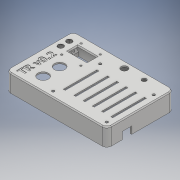
# Autodesk Inventor part: TestingRemoteHousing
Saved by Autodesk Inventor 2018.3 (Build 223284000, 284)
## iProperties
Created: 2019-03-25
Part Number: TestingRemoteHousing
Material: Generic
Document SubType Name: Modeling
Designer: matth
Density: 1 g/cm^3
Appearance: Default
Author: matth
Autodesk Inventor part; units mm, degrees
ref_plane "YZ Plane" through (0, 0, 0) normal (1, 0, 0) x (0, 1, 0)
ref_plane "XZ Plane" through (0, 0, 0) normal (0, 1, 0) x (-1, 0, 0)
ref_plane "XY Plane" through (0, 0, 0) normal (0, 0, 1) x (1, 0, 0)
sketch "Sketch1" plane through (0, 0, 0) normal (0, 0, 1) x (1, 0, 0)
  line L0 (-6.9712, 4.0639) -> (131.4288, 4.0639)
  line L1 (138.4288, -2.9361) -> (138.4288, -90.5361)
  line L2 (131.4288, -97.5361) -> (-6.9712, -97.5361)
  line L3 (-13.9712, -90.5361) -> (-13.9712, -2.9361)
  arc A0 (-6.9712, 4.0639) -> (-13.9712, -2.9361) centre (-6.9712, -2.9361) ccw
  arc A1 (-13.9712, -90.5361) -> (-6.9712, -97.5361) centre (-6.9712, -90.5361) ccw
  arc A2 (131.4288, -97.5361) -> (138.4288, -90.5361) centre (131.4288, -90.5361) ccw
  arc A3 (138.4288, -2.9361) -> (131.4288, 4.0639) centre (131.4288, -2.9361) ccw
  circle A4 centre (103.4288, -5.9361) radius 3.43
  circle A5 centre (130.4288, -89.5361) radius 2
  circle A6 centre (49.2288, -89.5361) radius 2
  circle A7 centre (49.2288, -18.3361) radius 2
  circle A8 centre (130.4288, -18.3361) radius 2
  circle A9 centre (8.0288, -5.9361) radius 1.5
  circle A10 centre (36.9848, -5.9361) radius 1.5
  circle A11 centre (8.0288, -35.4001) radius 1.5
  circle A12 centre (36.9848, -35.4001) radius 1.5
  circle A13 centre (22.0288, -52.5361) radius 8
  circle A14 centre (22.0288, -77.5361) radius 8
  line L4 (-7.9712, -7.9361) -> (0.2288, -7.9361)
  line L5 (0.2288, -7.9361) -> (0.2288, -16.1361)
  line L6 (0.2288, -16.1361) -> (-7.9712, -16.1361)
  line L7 (-7.9712, -16.1361) -> (-7.9712, -7.9361)
  line L8 (-7.9712, -20.8361) -> (0.2288, -20.8361)
  line L9 (0.2288, -20.8361) -> (0.2288, -29.0361)
  line L10 (0.2288, -29.0361) -> (-7.9712, -29.0361)
  line L11 (-7.9712, -29.0361) -> (-7.9712, -20.8361)
  circle A15 centre (73.4288, -5.9361) radius 5
  line L12 (8.0288, -26.0021) -> (36.9848, -26.0021)
  line L13 (36.9848, -26.0021) -> (36.9848, -11.0021)
  line L14 (36.9848, -11.0021) -> (8.0288, -11.0021)
  line L15 (8.0288, -11.0021) -> (8.0288, -26.0021)
  line L16 (54.5635, -28.5361) -> (57.5635, -28.5361)
  line L17 (57.5635, -28.5361) -> (57.5635, -79.5361)
  line L18 (57.5635, -79.5361) -> (54.5635, -79.5361)
  line L19 (54.5635, -79.5361) -> (54.5635, -28.5361)
  line L20 (70.5888, -79.5361) -> (73.5888, -79.5361)
  line L21 (73.5888, -79.5361) -> (73.5888, -28.5361)
  line L22 (73.5888, -28.5361) -> (70.5888, -28.5361)
  line L23 (70.5888, -28.5361) -> (70.5888, -79.5361)
  line L24 (84.5588, -28.5361) -> (87.5588, -28.5361)
  line L25 (87.5588, -28.5361) -> (87.5588, -79.5361)
  line L26 (87.5588, -79.5361) -> (84.5588, -79.5361)
  line L27 (84.5588, -79.5361) -> (84.5588, -28.5361)
  line L28 (98.5288, -28.5361) -> (101.5288, -28.5361)
  line L29 (101.5288, -28.5361) -> (101.5288, -79.5361)
  line L30 (101.5288, -79.5361) -> (98.5288, -79.5361)
  line L31 (98.5288, -79.5361) -> (98.5288, -28.5361)
  line L32 (112.4288, -28.5361) -> (115.4288, -28.5361)
  line L33 (115.4288, -28.5361) -> (115.4288, -79.5361)
  line L34 (115.4288, -79.5361) -> (112.4288, -79.5361)
  line L35 (112.4288, -79.5361) -> (112.4288, -28.5361)
  line L36 (126.4688, -28.5361) -> (129.4688, -28.5361)
  line L37 (129.4688, -28.5361) -> (129.4688, -79.5361)
  line L38 (129.4688, -79.5361) -> (126.4688, -79.5361)
  line L39 (126.4688, -79.5361) -> (126.4688, -28.5361)
  point P0 (0, 0)
  point P1 (138.4288, -97.5361)
  point P2 (138.4288, 4.0639)
  point P3 (-13.9712, -97.5361)
  dimension "d0" = 152.4
  dimension "d1" = 101.6
  dimension "d2" = 7
  dimension "d3" = 6.86
  dimension "d4" = 10
  dimension "d5" = 35
  dimension "d6" = 4
  dimension "d7" = 4
  dimension "d8" = 4
  dimension "d9" = 81.2
  dimension "d10" = 8
  dimension "d11" = 0
  dimension "d12" = 71.2
  dimension "d13" = 4
  dimension "d14" = 8
  dimension "d15" = 3
  dimension "d16" = 3
  dimension "d17" = 28.956
  dimension "d18" = 22
  dimension "d19" = 3
  dimension "d20" = 29.464
  dimension "d21" = 3
  dimension "d22" = 16
  dimension "d23" = 16
  dimension "d24" = 20
  dimension "d25" = 63.2
  dimension "d26" = 36
  dimension "d27" = 36
  dimension "d28" = 25
  dimension "d29" = 10
  dimension "d30" = 0
  dimension "d31" = 8.2
  dimension "d32" = 8.2
  dimension "d33" = 6
  dimension "d34" = 12
  dimension "d35" = 8.2
  dimension "d36" = 10
  dimension "d37" = 10
  dimension "d38" = 65
  dimension "d39" = 0
  dimension "d40" = 28.956
  dimension "d41" = 15
  dimension "d42" = 9.398
  dimension "d43" = 0
  dimension "d44" = 3
  dimension "d45" = 51
  dimension "d46" = 10.2
  dimension "d47" = 3
  dimension "d48" = 51
  dimension "d49" = 3
  dimension "d50" = 51
  dimension "d51" = 3
  dimension "d52" = 51
  dimension "d53" = 3
  dimension "d54" = 51
  dimension "d55" = 3
  dimension "d56" = 51
  dimension "d57" = 21.36
  dimension "d58" = 35.33
  dimension "d59" = 49.3
  dimension "d60" = 63.2
  dimension "d61" = 80.24
  dimension "d112" = 8.2
  dimension "d113" = 0
  constraints: 80 end point, 20 parallel, 16 centre point, 10 horizontal, 10 perpendicular, 10 point on line, 8 point on circle, 8 tangent, 3 equal radius
  measures "d0" distance of point (138.429, -97.536) point (-13.971, -97.536)
  measures "d1" distance of point (138.429, 4.064) point (138.429, -97.536)
  measures "d2" radius of A0
  measures "d3" diameter of A4
  measures "d4" distance from line of L0 A4.centre
  measures "d5" distance from line of L1 A4.centre
  measures "d6" diameter of A5
  measures "d7" diameter of A6
  measures "d8" diameter of A7
  measures "d9" distance of A6.centre A5.centre
  measures "d10" distance from line of L1 A5.centre
  measures "d11" horizontal distance of A7.centre A6.centre
  measures "d12" distance of A6.centre A7.centre
  measures "d13" diameter of A8
  measures "d14" distance from line of L2 A5.centre
  measures "d15" diameter of A9
  measures "d16" diameter of A10
  measures "d17" distance of A10.centre A9.centre
  measures "d18" distance from line of L3 A9.centre
  measures "d19" diameter of A11
  measures "d20" distance of A9.centre A11.centre
  measures "d21" diameter of A12
  measures "d22" diameter of A13
  measures "d23" diameter of A14
  measures "d24" distance from line of L2 A14.centre
  measures "d25" distance from line of A6.centre L3
  measures "d26" distance from line of L3 A14.centre
  measures "d27" distance from line of A13.centre L3
  measures "d28" distance of A14.centre A13.centre
  measures "d29" distance from line of L0 A9.centre
  measures "d30" vertical distance of A11.centre A12.centre
  measures "d31" distance of L5.end L6.end
  measures "d32" distance of L4.end L5.end
  measures "d33" distance between parallel lines of L3 L7
  measures "d34" distance between parallel lines of L0 L4
  measures "d35" distance of L8.end L9.end
  measures "d36" diameter of A15
  measures "d37" distance from line of A15.centre L0
  measures "d38" distance from line of L1 A15.centre
  measures "d39" vertical distance of A8.centre A7.centre
  measures "d40" distance of L14.end L13.end
  measures "d41" distance of L12.end L13.end
  measures "d42" distance from line of L12 A11.centre
  measures "d43" distance from line of A10.centre L13
  measures "d44" distance of L17.end L18.end
  measures "d45" distance of L16.end L17.end
  measures "d46" distance from line of A7.centre L16
  measures "d47" distance of L22.end L21.end
  measures "d48" distance of L21.end L20.end
  measures "d49" distance of L25.end L26.end
  measures "d50" distance of L24.end L25.end
  measures "d51" distance of L29.end L30.end
  measures "d52" distance of L28.end L29.end
  measures "d53" distance of L33.end L34.end
  measures "d54" distance of L32.end L33.end
  measures "d55" distance of L37.end L38.end
  measures "d56" distance of L36.end L37.end
  measures "d57" distance from line of L23 A7.centre
  measures "d58" distance from line of A7.centre L27
  measures "d59" distance from line of L31 A7.centre
  measures "d60" distance from line of A7.centre L35
  measures "d61" distance from line of A7.centre L37
  measures "d112" distance of L9.end L10.end
  measures "d113" distance between parallel lines of L7 L11
extrude "Extrusion1" add sketch "Sketch1" along normal blind 2
chamfer "Chamfer1" distance 1 distance2 2 1 edges at (36.9848, -18.5021, 2) measured on face at (37.4848, -18.5021, 2)
chamfer "Chamfer2" distance 1 distance2 2 2 edges at (37.4848, -11.0021, 2) (22.5068, -11.0021, 2) measured on face at (37.4848, -10.5021, 2) measured on face at (22.5068, -10.5021, 2)
chamfer "Chamfer3" distance 1 distance2 2 2 edges at (8.0288, -10.5021, 2) (8.0288, -18.5021, 2) measured on face at (7.5288, -18.5021, 2) measured on face at (7.5288, -10.5021, 2)
chamfer "Chamfer4" distance 1 distance2 2 3 edges at (7.5289, -26.0021, 2) (22.5068, -26.0021, 2) (37.4848, -26.0021, 2) measured on face at (37.4848, -26.5021, 2) measured on face at (22.5068, -26.5021, 2) measured on face at (7.5289, -26.5021, 2)
chamfer "Chamfer5" distance 1 distance2 2 8 edges at (-13.9712, -46.7361, 2) (-11.9209, -95.4858, 2) (62.2288, -97.5361, 2) (136.3786, -95.4858, 2) (138.4288, -46.7361, 2) (136.3786, 2.0136, 2) (62.2288, 4.0639, 2) (-11.9209, 2.0136, 2) measured on face at (136.025, 1.6601, 2) measured on face at (62.2288, -97.0361, 2) measured on face at (62.2288, 3.5639, 2) measured on face at (-11.5674, -95.1323, 2) measured on face at (-11.5674, 1.6601, 2) measured on face at (137.9288, -46.7361, 2) measured on face at (136.025, -95.1323, 2) measured on face at (-13.4712, -46.7361, 2)
sketch "Sketch2" plane through (0, 0, 0) normal (0, 0, -1) x (-1, 0, 0)
  line L0 (6.9712, -97.5361) -> (-131.4288, -97.5361) projected
  arc A0 (6.9712, -97.5361) -> (13.9712, -90.5361) centre (6.9712, -90.5361) ccw projected
  line L1 (13.9712, -2.9361) -> (13.9712, -90.5361) projected
  arc A1 (13.9712, -2.9361) -> (6.9712, 4.0639) centre (6.9712, -2.9361) ccw projected
  line L2 (-131.4288, 4.0639) -> (6.9712, 4.0639) projected
  arc A2 (-131.4288, 4.0639) -> (-138.4288, -2.9361) centre (-131.4288, -2.9361) ccw projected
  line L3 (-138.4288, -90.5361) -> (-138.4288, -2.9361) projected
  arc A3 (-138.4288, -90.5361) -> (-131.4288, -97.5361) centre (-131.4288, -90.5361) ccw projected
  line L4 (-131.4288, -95.5361) -> (6.9712, -95.5361)
  arc A4 (6.9712, -95.5361) -> (11.9712, -90.5361) centre (6.9712, -90.5361) ccw
  line L5 (11.9712, -90.5361) -> (11.9712, -2.9361)
  arc A5 (11.9712, -2.9361) -> (6.9712, 2.0639) centre (6.9712, -2.9361) ccw
  line L6 (6.9712, 2.0639) -> (-131.4288, 2.0639)
  arc A6 (-131.4288, 2.0639) -> (-136.4288, -2.9361) centre (-131.4288, -2.9361) ccw
  line L7 (-136.4288, -2.9361) -> (-136.4288, -90.5361)
  arc A7 (-136.4288, -90.5361) -> (-131.4288, -95.5361) centre (-131.4288, -90.5361) ccw
  point P0 (0, 0)
  dimension "d79" = 2
  constraints: 8 end point, 8 point on circle, 4 centre point, 7 other
  measures "d79" distance between parallel lines of L0 L4
extrude "Extrusion2" add sketch "Sketch2" along normal blind 25
sketch "Sketch3" plane through (0, 0, -25) normal (0, 0, -1) x (-1, 0, 0)
  line L0 (-131.4288, 2.0639) -> (6.9712, 2.0639) projected
  arc A0 (-131.4288, 2.0639) -> (-136.4288, -2.9361) centre (-131.4288, -2.9361) ccw projected
  line L1 (-136.4288, -90.5361) -> (-136.4288, -2.9361) projected
  arc A1 (-136.4288, -90.5361) -> (-131.4288, -95.5361) centre (-131.4288, -90.5361) ccw projected
  line L2 (6.9712, -95.5361) -> (-131.4288, -95.5361) projected
  arc A2 (6.9712, -95.5361) -> (11.9712, -90.5361) centre (6.9712, -90.5361) ccw projected
  line L3 (11.9712, -2.9361) -> (11.9712, -90.5361) projected
  arc A3 (11.9712, -2.9361) -> (6.9712, 2.0639) centre (6.9712, -2.9361) ccw projected
  line L4 (3.9712, -5.9361) -> (-128.4288, -5.9361)
  line L5 (-128.4288, -5.9361) -> (-128.4288, -87.5361)
  line L6 (-128.4288, -87.5361) -> (3.9712, -87.5361)
  line L7 (3.9712, -87.5361) -> (3.9712, -5.9361)
  line L8 (-128.4288, -5.9361) -> (-128.4288, 2.0639)
  line L9 (-128.4288, -5.9361) -> (-136.4288, -5.9361)
  line L10 (3.9712, -5.9361) -> (3.9712, 2.0639)
  line L11 (3.9712, -5.9361) -> (11.9712, -5.9361)
  line L12 (-128.4288, -87.5361) -> (11.9712, -87.5361)
  line L13 (11.9712, -90.5361) -> (11.9712, -2.9361) projected
  line L14 (3.9712, -5.9361) -> (3.9712, -95.5361)
  line L15 (-131.4288, -95.5361) -> (6.9712, -95.5361) projected
  line L16 (-128.4288, -87.5361) -> (-136.4288, -87.5361)
  line L17 (-136.4288, -2.9361) -> (-136.4288, -90.5361) projected
  line L18 (-128.4288, -87.5361) -> (-128.4288, -95.5361)
  point P0 (0, 0)
  dimension "d82" = 8
  constraints: 24 end point, 12 point on line, 4 perpendicular, 2 vertical, 3 other
  measures "d82" distance between parallel lines of L0 L4
extrude "Extrusion3" add sketch "Sketch3" against normal blind 14 contours L0 L8 L9 L1 A0 | L0 A3 L3 L11 L10 | L11 L3 L12 L7 | L18 L2 A1 L1 L16 | L12 L3 A2 L2 L14
chamfer "Chamfer6" distance 8 angle 45 3 edges at (128.4288, -91.5361, -11) (128.4288, -1.9361, -11) (-3.9712, -46.7361, -11)
sketch "Sketch4" plane through (0, 0, -25) normal (0, 0, -1) x (-1, 0, 0)
  circle A0 centre (-131.4288, -90.5361) radius 1.75
  line L0 (-138.4288, -2.9361) -> (-138.4288, -90.5361) projected
  line L1 (-131.4288, -97.5361) -> (6.9712, -97.5361) projected
  circle A1 centre (-131.4288, -2.9361) radius 1.75
  line L2 (6.9712, 4.0639) -> (-131.4288, 4.0639) projected
  circle A2 centre (6.9712, -2.9361) radius 1.75
  line L3 (13.9712, -90.5361) -> (13.9712, -2.9361) projected
  circle A3 centre (6.9712, -90.5361) radius 1.75
  point P0 (0, 0)
  dimension "d88" = 3.5
  dimension "d89" = 7
  dimension "d90" = 7
  dimension "d91" = 3.5
  dimension "d92" = 7
  dimension "d93" = 7
  dimension "d94" = 3.5
  dimension "d95" = 7
  dimension "d96" = 7
  dimension "d97" = 3.5
  dimension "d98" = 7
  dimension "d99" = 7
  constraints: 4 centre point
  measures "d88" diameter of A0
  measures "d89" distance from line of L0 A0.centre
  measures "d90" distance from line of L1 A0.centre
  measures "d91" diameter of A1
  measures "d92" distance from line of L0 A1.centre
  measures "d93" distance from line of L2 A1.centre
  measures "d94" diameter of A2
  measures "d95" distance from line of L3 A2.centre
  measures "d96" distance from line of L2 A2.centre
  measures "d97" diameter of A3
  measures "d98" distance from line of L1 A3.centre
  measures "d99" distance from line of L3 A3.centre
extrude "Extrusion4" cut sketch "Sketch4" against normal blind 12
sketch "Sketch5" plane through (138.4288, -90.5361, 0) normal (1, 0, 0) x (0, 0, -1)
  line L0 (-2, -1) -> (-2, 3) projected
  line L1 (-2, 70.2) -> (-2, 74.2) projected
  line L2 (14, 16.5909) -> (25, 16.5909)
  line L3 (25, 16.5909) -> (25, 30.5909)
  line L4 (25, 30.5909) -> (14, 30.5909)
  line L5 (14, 30.5909) -> (14, 16.5909)
  line L6 (-2, 87.6) -> (-2, 0) projected
  line L7 (25, 87.6) -> (25, 0) projected
  point P0 (0, 90.5361)
  point P1 (-2, 1)
  point P2 (-2, 72.2)
  dimension "d102" = 11
  dimension "d103" = 14
  dimension "d105" = 0
  constraints: 8 end point, 2 midpoint, 2 parallel, 1 horizontal, 1 perpendicular
  measures "d102" distance of L4.end L3.end
  measures "d103" distance of L3.end L2.end
  measures "d105" distance between parallel lines of L7 L3
extrude "Extrusion5" cut sketch "Sketch5" against normal blind 10
sketch "Sketch6" plane through (0, 0, -25) normal (0, 0, -1) x (-1, 0, 0)
  line L0 (3.9712, 2.0639) -> (3.9712, -95.5361) projected
  line L1 (13.9712, -90.5361) -> (13.9712, -2.9361) projected
  line L2 (3.9712, -87.5361) -> (11.9712, -87.5361)
  line L3 (11.9712, -90.5361) -> (11.9712, -2.9361) projected
  line L4 (11.9712, -5.9361) -> (3.9712, -5.9361)
  line L5 (-128.4288, -87.5361) -> (-136.4288, -87.5361) projected
  line L6 (-136.4288, -5.9361) -> (-128.4288, -5.9361) projected
  line L7 (3.9712, -87.5361) -> (3.9712, -5.9361)
  line L8 (11.9712, -5.9361) -> (11.9712, -87.5361)
  point P0 (0, 0)
  dimension "d108" = 0
  dimension "d109" = 0
  constraints: 8 end point, 3 point on line, 1 collinear, 1 horizontal, 1 perpendicular, 1 vertical
  measures "d108" distance between parallel lines of L5 L2
  measures "d109" distance between parallel lines of L6 L4
extrude "Extrusion6" cut sketch "Sketch6" against normal up to surface (25 mm away)
sketch "Sketch7" plane through (0, 0, 2) normal (0, 0, 1) x (1, 0, 0)
  line L0 (-7.9712, -7.9361) -> (0.2288, -7.9361) projected
  line L1 (-7.9712, -16.1361) -> (-7.9712, -7.9361) projected
  line L2 (0.2288, -7.9361) -> (0.2288, -16.1361) projected
  line L3 (0.2288, -16.1361) -> (-7.9712, -16.1361) projected
  line L4 (-7.9712, -20.8361) -> (0.2288, -20.8361) projected
  line L5 (-7.9712, -29.0361) -> (-7.9712, -20.8361) projected
  line L6 (0.2288, -29.0361) -> (-7.9712, -29.0361) projected
  line L7 (0.2288, -20.8361) -> (0.2288, -29.0361) projected
  circle A0 centre (-3.8712, -12.0361) radius 4.1
  circle A1 centre (-3.8712, -24.9361) radius 4.1
  point P0 (0, 0)
  constraints: 2 centre point
extrude "Extrusion7" add sketch "Sketch7" against normal blind 0.5 contours L0 A0 L1 | L0 L2 A0 | A0 L3 L1 | L2 L3 A0 | L4 A1 L5 | L4 L7 A1 | A1 L6 L5 | L7 L6 A1
chamfer "Chamfer7" distance 0.2 angle 45 8 edges at (-3.8712, -29.0361, 0) (0.2288, -24.9361, 0) (-7.9712, -24.9361, 0) (-3.8712, -20.8361, 0) (-3.8712, -16.1361, 0) (0.2288, -12.0361, 0) (-3.8712, -7.9361, 0) (-7.9712, -12.0361, 0)
sketch "Sketch8" plane through (0, 0, 2) normal (0, 0, 1) x (1, 0, 0)
  line L0 (-5.4333, -90.7908) -> (-5.4333, -38.3713) construction
  line L1 (-5.4333, -38.3713) -> (35.6473, -38.3713) construction
  line L2 (35.6473, -38.3713) -> (35.6473, -90.7908) construction
  line L3 (35.6473, -90.7908) -> (-5.4333, -90.7908) construction
  line L4 (4.7693, -87.833) -> (-3.3263, -87.833)
  line L5 (-3.3263, -87.833) -> (-3.3263, -90.7908)
  line L6 (-3.3263, -90.7908) -> (-5.2307, -90.7908)
  line L7 (-5.2307, -90.7908) -> (-5.2307, -82.3629)
  line L8 (-5.2307, -82.3629) -> (-3.3263, -82.3629)
  line L9 (-3.3263, -82.3629) -> (-3.3263, -85.3208)
  line L10 (-3.3263, -85.3208) -> (4.7693, -85.3208)
  line L11 (4.7693, -85.3208) -> (4.7693, -87.833)
  line L12 (4.7693, -72.0955) -> (4.7693, -75.1506)
  line L13 (4.7693, -75.1506) -> (1.0983, -77.9302)
  line L14 (1.0983, -77.9302) -> (1.0983, -78.8378)
  line L15 (1.0983, -78.8378) -> (4.7693, -78.8378)
  line L16 (4.7693, -78.8378) -> (4.7693, -81.3338)
  line L17 (4.7693, -81.3338) -> (-5.2307, -81.3338)
  line L18 (-5.2307, -81.3338) -> (-5.2307, -77.3143)
  spline S0 degree 2 poles (-5.2307, -77.3143) (-5.2307, -76.4796) (-5.02, -75.2479) (-4.6958, -74.7211) knots 0 0 0 1 2 2 2
  spline S1 degree 2 poles (-4.6958, -74.7211) (-4.3555, -74.1863) (-3.2939, -73.5542) (-2.4835, -73.5542) knots 0 0 0 1 2 2 2
  spline S2 degree 2 poles (-2.4835, -73.5542) (-1.3409, -73.5542) (0.0935, -74.5915) (0.5148, -75.4586) knots 0 0 0 1 2 2 2
  line L19 (0.5148, -75.4586) -> (4.7693, -72.0955)
  spline S3 degree 2 poles (-2.1675, -76.1312) (-2.5484, -76.1312) (-3.0913, -76.4229) (-3.2372, -76.7552) knots 0 0 0 1 2 2 2
  spline S4 degree 2 poles (-3.2372, -76.7552) (-3.3344, -76.9902) (-3.3911, -77.5655) (-3.3911, -77.995) knots 0 0 0 1 2 2 2
  line L20 (-3.3911, -77.995) -> (-3.3911, -78.8378)
  line L21 (-3.3911, -78.8378) -> (-0.7007, -78.8378)
  line L22 (-0.7007, -78.8378) -> (-0.7007, -78.1166)
  spline S5 degree 2 poles (-0.7007, -78.1166) (-0.7007, -77.5979) (-0.8304, -76.8605) (-1.033, -76.6093) knots 0 0 0 1 2 2 2
  spline S6 degree 2 poles (-1.033, -76.6093) (-1.2275, -76.3662) (-1.7461, -76.1312) (-2.1675, -76.1312) knots 0 0 0 1 2 2 2
  line L23 (-2.7753, -60.4018) -> (4.7693, -63.1085)
  line L24 (4.7693, -63.1085) -> (4.7693, -65.6774)
  line L25 (4.7693, -65.6774) -> (-2.7753, -68.3597)
  line L26 (-2.7753, -68.3597) -> (-2.7753, -65.8881)
  line L27 (-2.7753, -65.8881) -> (2.2085, -64.3484)
  line L28 (2.2085, -64.3484) -> (-2.7753, -62.8249)
  line L29 (-2.7753, -62.8249) -> (-2.7753, -60.4018)
  spline S7 degree 2 poles (-0.2307, -52.1685) (1.0659, -52.1685) (3.0108, -52.5817) (3.6672, -53.0437) knots 0 0 0 1 2 2 2
  spline S8 degree 2 poles (3.6672, -53.0437) (4.3155, -53.4975) (4.98, -54.9642) (4.98, -56.0177) knots 0 0 0 1 2 2 2
  spline S9 degree 2 poles (4.98, -56.0177) (4.98, -57.0793) (4.3155, -58.538) (3.651, -58.9999) knots 0 0 0 1 2 2 2
  spline S10 degree 2 poles (3.651, -58.9999) (2.9946, -59.4618) (1.0659, -59.8751) (-0.2307, -59.8751) knots 0 0 0 1 2 2 2
  spline S11 degree 2 poles (-0.2307, -59.8751) (-1.5597, -59.8751) (-3.4398, -59.4618) (-4.1205, -58.9918) knots 0 0 0 1 2 2 2
  spline S12 degree 2 poles (-4.1205, -58.9918) (-4.785, -58.5218) (-5.4333, -57.0388) (-5.4333, -56.0177) knots 0 0 0 1 2 2 2
  spline S13 degree 2 poles (-5.4333, -56.0177) (-5.4333, -54.9399) (-4.7526, -53.4975) (-4.08, -53.0356) knots 0 0 0 1 2 2 2
  spline S14 degree 2 poles (-4.08, -53.0356) (-3.4236, -52.5817) (-1.4868, -52.1685) (-0.2307, -52.1685) knots 0 0 0 1 2 2 2
  spline S15 degree 2 poles (-0.2307, -54.6887) (-2.0864, -54.6887) (-3.5856, -55.2965) (-3.5856, -56.0177) knots 0 0 0 1 2 2 2
  spline S16 degree 2 poles (-3.5856, -56.0177) (-3.5856, -56.739) (-2.0864, -57.3548) (-0.2226, -57.3548) knots 0 0 0 1 2 2 2
  spline S17 degree 2 poles (-0.2226, -57.3548) (1.6089, -57.3548) (3.1324, -56.739) (3.1324, -56.0177) knots 0 0 0 1 2 2 2
  spline S18 degree 2 poles (3.1324, -56.0177) (3.1324, -55.3046) (1.6089, -54.6887) (-0.2307, -54.6887) knots 0 0 0 1 2 2 2
  line L30 (4.7693, -48.3111) -> (4.7693, -50.6855)
  line L31 (4.7693, -50.6855) -> (2.1275, -50.6855)
  line L32 (2.1275, -50.6855) -> (2.1275, -48.3111)
  line L33 (2.1275, -48.3111) -> (4.7693, -48.3111)
  line L34 (4.7693, -38.9837) -> (4.7693, -46.3338)
  line L35 (4.7693, -46.3338) -> (3.1405, -46.3338)
  spline S19 degree 2 poles (3.1405, -46.3338) (2.3949, -45.4018) (1.0821, -43.9108) (0.4905, -43.3516) knots 0 0 0 1 2 2 2
  spline S20 degree 2 poles (0.4905, -43.3516) (-0.2793, -42.6142) (-1.4544, -41.9578) (-2.0702, -41.9578) knots 0 0 0 1 2 2 2
  spline S21 degree 2 poles (-2.0702, -41.9578) (-2.7672, -41.9578) (-3.5127, -42.7924) (-3.5127, -43.538) knots 0 0 0 1 2 2 2
  spline S22 degree 2 poles (-3.5127, -43.538) (-3.5127, -43.9189) (-3.3263, -44.5996) (-3.1805, -44.948) knots 0 0 0 1 2 2 2
  spline S23 degree 2 poles (-3.1805, -44.948) (-3.0265, -45.2884) (-2.7023, -45.7746) (-2.6213, -45.8962) knots 0 0 0 1 2 2 2
  line L36 (-2.6213, -45.8962) -> (-2.6213, -46.0907)
  line L37 (-2.6213, -46.0907) -> (-4.8012, -46.0907)
  spline S24 degree 2 poles (-4.8012, -46.0907) (-5.0038, -45.6693) (-5.4252, -43.8702) (-5.4252, -43.0356) knots 0 0 0 1 2 2 2
  spline S25 degree 2 poles (-5.4252, -43.0356) (-5.4252, -41.2527) (-3.8369, -39.4213) (-2.4025, -39.4213) knots 0 0 0 1 2 2 2
  spline S26 degree 2 poles (-2.4025, -39.4213) (-1.5192, -39.4213) (0.1826, -40.256) (1.155, -41.2203) knots 0 0 0 1 2 2 2
  spline S27 degree 2 poles (1.155, -41.2203) (1.7547, -41.8281) (2.6866, -42.9707) (2.8811, -43.2219) knots 0 0 0 1 2 2 2
  line L38 (2.8811, -43.2219) -> (2.8811, -38.9837)
  line L39 (2.8811, -38.9837) -> (4.7693, -38.9837)
  point P0 (0, 0)
  constraints: 2 other
emboss "Emboss1" sketch "Sketch8" operation cut depth 0.5 direction (0, 0, -1)
equation "\"d27\" = d26"
body "Solid1"
